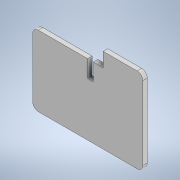
# Autodesk Inventor part: pcb_balun_bottom
Saved by Autodesk Inventor 2020.2 (Build 242310000, 310)
## iProperties
Created: 2020-09-26
Part Number: pcb_balun_bottom
Material: Generic
Document SubType Name: Modeling
Designer: Krishna Makhija
Density: 1 g/cm^3
Appearance: Default
Author: Krishna Makhija
Autodesk Inventor part; units mm, degrees
ref_plane "YZ Plane" through (0, 0, 0) normal (1, 0, 0) x (0, 1, 0)
ref_plane "XZ Plane" through (0, 0, 0) normal (0, 1, 0) x (-1, 0, 0)
ref_plane "XY Plane" through (0, 0, 0) normal (0, 0, 1) x (1, 0, 0)
sketch "Sketch6" plane through (0, 0, 0) normal (0, 0, 1) x (1, 0, 0)
  line L0 (19.5, -12.4999) -> (-19.5, -12.4999)
  line L1 (-19.5, -12.4999) -> (-19.5, 12.4999)
  line L2 (19.5, 12.4999) -> (19.5, -12.4999)
  line L3 (19.5, -12.4999) -> (-19.5, 12.4999) construction
  line L4 (-19.5, -12.4999) -> (19.5, 12.4999) construction
  line L5 (5.4997, 12.4999) -> (5.4997, 17.5003)
  line L6 (5.4997, 17.5003) -> (19.5, 17.5003)
  line L7 (19.5, 17.5003) -> (19.5, 12.4999)
  line L8 (1.9998, 6.5001) -> (0.0002, 6.5001)
  line L9 (0.0002, 6.5001) -> (0.0002, 12.4999)
  line L10 (1.9998, 12.4999) -> (1.9998, 6.5001)
  line L11 (1.9998, 6.5001) -> (0.0002, 12.4999) construction
  line L12 (0.0002, 6.5001) -> (1.9998, 12.4999) construction
  line L13 (-19.5, 12.4999) -> (0.0002, 12.4999)
  line L14 (1.9998, 12.4999) -> (5.4997, 12.4999)
  constraints: 30 end point, 3 parallel, 3 perpendicular, 2 horizontal, 1 collinear
extrude "Extrusion5" add sketch "Sketch6" along normal blind 1.6
fillet "Fillet5" radius 2 4 edges at (19.5, 17.5003, 0.8) (-19.5, 12.4999, 0.8) (-19.5, -12.4999, 0.8) (19.5, -12.4999, 0.8)
body "Solid5"
